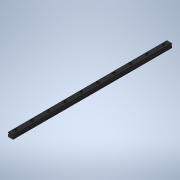
# Autodesk Inventor part: SSEB6-145-B3_r
Saved by Autodesk Inventor 2021 (Build 250183000, 183)
## iProperties
Created: 2025-06-10
Part Number: SSEB6-145-B3_r
Material: Generic
Catalog Web Link: www.cadenas.de
Description: SSEB, SSEB-MX, SSEBV, SSEBV-MX, SSE2B, SSE2B-MX, SSE2BV, SSE2BV-MX, SSEBL, SSEBL-MX, SSEBLV, SSEBLV-MX, SSE2BL, SSE2BL-MX, SSE2BLV, SSE2BLV-MX, SEB, SEBV, SE2B, SE2BV, SEBL, SEBLV, SE2BL, SE2BLV_rail-Miniature Linear Guides - Short Block, Standard Preload - High/Precision Grade
Vendor: MISUMI
Document SubType Name: Modeling
Designer: psAdmin
Manufacturer: MISUMI
Mass: 2.44458 g
Surface Area: 32.5102 cm^2
Volume: 2.44458 cm^3
Density: 1 g/cm^3
Appearance: PSOLRGB-175-175-175
Category: PARTsolutions
Company: MISUMI
Title: SSEB6-145-B3
Author: Cadenas PARTsolutions
Comments: Miniature Linear Guides - Short Block, Standard Preload - High/Precision Grade
PSOL_IDENT_0: {$CADENAS_DATA/23d-libs/misumi/metric/06_linear_guides/seb_series/seb_rail.prj},398 {VTYP=3D},{NB=SS
PSOL_IDENT_1: EB6-145-B3_r},{LINA=SSEB6-145-B3},{NN=SSEB, SSEB-MX, SSEBV, SSEBV-MX, SSE2B, SSE2B-MX, SSE2BV, SSE2B
PSOL_IDENT_2: V-MX, SSEBL, SSEBL-MX, SSEBLV, SSEBLV-MX, SSE2BL, SSE2BL-MX, SSE2BLV, SSE2BLV-MX, SEB, SEBV, SE2B, S
PSOL_IDENT_3: E2BV, SEBL, SEBLV, SE2BL, SE2BLV_rail},{DATE=17.02.2022 00:32:34},{GEOMDATE=21.01.2022 00:02:30},{VE
PSOL_IDENT_4: RSION=},{LINEID=90},{WBVAR=TS,ST,MAT,MX,NOB,LT,LS,ALT1,ALT2,ALT4},{WBNUMERIC=LS}  {NB=SSEB6-145-B3_r
PSOL_IDENT_5: },{LINA=SSEB6-145-B3},{KT=DUMMY},{PN=SSEB6-145-B3},{RT=B},{TS=},{TS1=  '','Advanced'  },{TYPE=SSEB},
PSOL_IDENT_6: {ST=S},{MAT=S},{MX=},{MXALG= '','w/o MX(Lubrication unit)' },{NOB=},{H=6},{LT=Selectable},{LTALG='Se
PSOL_IDENT_7: lectable','Selectable','Configurable','Configurable'},{LS=145},{W=12},{L1=17.4},{B=8},{C=0},{S=M2X1.
PSOL_IDENT_8: 5},{L2=9.7},{K=4.5},{CBB=0.3},{W1=5},{W2=3.5},{H1=4.0},{CAA=0.3},{DD1DD2HH=2.4x3.5x1},{F=15},{G=5.0}
PSOL_IDENT_9: ,{DD1=2.400},{DD2=3.500},{HH=1.000},{ALT1=},{ALT1ALG='', 'w/o MC (Tapped Holes)', '-MC', 'with MC (T
PSOL_IDENT_10: apped Holes)'},{MC=M2.6},{MC1=2.6},{ALT2=},{ALT2L=0.0},{ALT2N=0},{M=10},{LL=},{L0=25,40,55,70,85,100
PSOL_IDENT_11: ,115,130,145},{REC1=   '','Not applicable'    },{ST1='S', 'w/o Surface Treatment'},{MAT2='S','Stainl
PSOL_IDENT_12: ess Steel'},{NL=32.867},{ALT4=-B3},{ALT4ALG= '','w/o (Additional Blocks)','-B3','with B3(3-Block Typ
PSOL_IDENT_13: e (Adds 2 blocks.))','-B4','with B4(4-Block Type (Adds 3 blocks.))' },{CA1=0.3},{CA2=0.3},{VA1=1.5},
PSOL_IDENT_14: {HA1=1.0},{HA2=5.1372},{WA1=1.2167},{WA2=0.5},{RA1=1.00},{POIA1=-0.1473},{NA1=9},{LSC=6.0},{MS=2.0}
NB: SSEB6-145-B3_r
NN: SSEB, SSEB-MX, SSEBV, SSEBV-MX, SSE2B, SSE2B-MX, SSE2BV, SSE2BV-MX, SSEBL, SSEBL-MX, SSEBLV, SSEBLV-MX, SSE2BL, SSE2BL-MX, SSE2BLV, SSE2BLV-MX, SEB, SEBV, SE2B, SE2BV, SEBL, SEBLV, SE2BL, SE2BLV_rail
NT: Miniature Linear Guides - Short Block, Standard Preload - High/Precision Grade
NBSYN: $PN._r
LINA: SSEB6-145-B3
CATALOG: Misumi
PN: SSEB6-145-B3
TS: Advanced
ST: w/o Surface Treatment
MAT: Stainless Steel
MX: w/o MX(Lubrication unit)
NOB: 1
H: 6
LT: Selectable
LS: 145
W: 12
L1: 17.4
B: 8
C: 0
S: M2X1.5
L2: 9.7
K: 4.5
CBB: 0.3
W1: 5
W2: 3.5
H1: 4
CAA: 0.3
DD1DD2HH: 2.4x3.5x1
F: 15
G: 5
ALT1: w/o MC (Tapped Holes)
ALT2: Not applicable
ALT4: with B3(3-Block Type (Adds 2 blocks.))
NA1: 9
SUPPLIER: MISUMI
ARTICLENO: SSEB6-145-B3_r
BOMINFO: SSEB6-145-B3
CREATOR: CADENAS GmbH
Autodesk Inventor part; units mm, degrees
sketch "Sketch_12" plane through (0, 0, 0) normal (0, 0, 1) x (1, 0, 0)
  line L0 (-2.5, 3.7) -> (-2.5, 3.1084)
  line L1 (-2.5, 3.1084) -> (-2.3242, 3.0098)
  arc A0 (-2.1007, 2.75) -> (-2.3242, 3.0098) centre (-2.5686, 2.5736) ccw
  line L2 (-2.1007, 2.75) -> (-1.5, 2.75)
  line L3 (-1.5, 2.75) -> (-1.5, 2.25)
  line L4 (-1.5, 2.25) -> (-2.1007, 2.25)
  arc A1 (-2.3242, 1.9902) -> (-2.1007, 2.25) centre (-2.5686, 2.4264) ccw
  line L5 (-2.3242, 1.9902) -> (-2.5, 1.8917)
  line L6 (-2.5, 1.8917) -> (-2.5, 0.3)
  line L7 (-2.5, 0.3) -> (-2.2, 0)
  line L8 (-2.2, 0) -> (2.2, 0)
  line L9 (2.2, 0) -> (2.5, 0.3)
  line L10 (2.5, 0.3) -> (2.5, 1.8917)
  line L11 (2.5, 1.8917) -> (2.3242, 1.9902)
  arc A2 (2.1007, 2.25) -> (2.3242, 1.9902) centre (2.5686, 2.4263) ccw
  line L12 (2.1007, 2.25) -> (1.5, 2.25)
  line L13 (1.5, 2.25) -> (1.5, 2.75)
  line L14 (1.5, 2.75) -> (2.1007, 2.75)
  arc A3 (2.3242, 3.0098) -> (2.1007, 2.75) centre (2.5686, 2.5737) ccw
  line L15 (2.3242, 3.0098) -> (2.5, 3.1084)
  line L16 (2.5, 3.1084) -> (2.5, 3.7)
  line L17 (2.5, 3.7) -> (2.2, 4)
  line L18 (2.2, 4) -> (-2.2, 4)
  line L19 (-2.2, 4) -> (-2.5, 3.7)
  constraints: 40 end point, 8 point on circle, 4 centre point
extrude "Extrusion1" add sketch "Sketch_12" along normal mid plane 145
sketch "Sketch2" plane through (-2.2, 4, 72.5) normal (0, 1, 0) x (1, 0, 0)
  point P0 (2.2, 140)
hole "Hole1" at (0, 4, -67.5) direction (0, -1, 0) diameter 2.4 depth 4 counterbore diameter 3.5 counterbore depth 1
pattern_linear "Rectangular Pattern1" count 10 spacing 15 along (0, 0, 1) of "Hole1"
ref_plane "rail_to_adjusting_block_XY" through (0, 0, -67.5) normal (0, 1, 0) x (1, 0, 0)
ref_plane "rail_to_adjusting_block_YZ" through (0, 0, -67.5) normal (1, 0, 0) x (0, 0, -1)
ref_plane "rail_to_adjusting_block_ZX" through (0, 0, -67.5) normal (0, 0, -1) x (0, 1, 0)
ref_plane "screw_1_XY" through (0, 3, 67.5) normal (0, -1, 0) x (1, 0, 0)
ref_plane "screw_1_YZ" through (0, 3, 67.5) normal (1, 0, 0) x (0, 0, 1)
ref_plane "screw_1_ZX" through (0, 3, 67.5) normal (0, 0, 1) x (0, -1, 0)
ref_plane "screw_10_XY" through (0, 3, -67.5) normal (0, -1, 0) x (1, 0, 0)
ref_plane "screw_10_YZ" through (0, 3, -67.5) normal (1, 0, 0) x (0, 0, 1)
ref_plane "screw_10_ZX" through (0, 3, -67.5) normal (0, 0, 1) x (0, -1, 0)
ref_plane "screw_2_XY" through (0, 3, 52.5) normal (0, -1, 0) x (1, 0, 0)
ref_plane "screw_2_YZ" through (0, 3, 52.5) normal (1, 0, 0) x (0, 0, 1)
ref_plane "screw_2_ZX" through (0, 3, 52.5) normal (0, 0, 1) x (0, -1, 0)
ref_plane "screw_3_XY" through (0, 3, 37.5) normal (0, -1, 0) x (1, 0, 0)
ref_plane "screw_3_YZ" through (0, 3, 37.5) normal (1, 0, 0) x (0, 0, 1)
ref_plane "screw_3_ZX" through (0, 3, 37.5) normal (0, 0, 1) x (0, -1, 0)
ref_plane "screw_4_XY" through (0, 3, 22.5) normal (0, -1, 0) x (1, 0, 0)
ref_plane "screw_4_YZ" through (0, 3, 22.5) normal (1, 0, 0) x (0, 0, 1)
ref_plane "screw_4_ZX" through (0, 3, 22.5) normal (0, 0, 1) x (0, -1, 0)
ref_plane "screw_5_XY" through (0, 3, 7.5) normal (0, -1, 0) x (1, 0, 0)
ref_plane "screw_5_YZ" through (0, 3, 7.5) normal (1, 0, 0) x (0, 0, 1)
ref_plane "screw_5_ZX" through (0, 3, 7.5) normal (0, 0, 1) x (0, -1, 0)
ref_plane "screw_6_XY" through (0, 3, -7.5) normal (0, -1, 0) x (1, 0, 0)
ref_plane "screw_6_YZ" through (0, 3, -7.5) normal (1, 0, 0) x (0, 0, 1)
ref_plane "screw_6_ZX" through (0, 3, -7.5) normal (0, 0, 1) x (0, -1, 0)
ref_plane "screw_7_XY" through (0, 3, -22.5) normal (0, -1, 0) x (1, 0, 0)
ref_plane "screw_7_YZ" through (0, 3, -22.5) normal (1, 0, 0) x (0, 0, 1)
ref_plane "screw_7_ZX" through (0, 3, -22.5) normal (0, 0, 1) x (0, -1, 0)
ref_plane "screw_8_XY" through (0, 3, -37.5) normal (0, -1, 0) x (1, 0, 0)
ref_plane "screw_8_YZ" through (0, 3, -37.5) normal (1, 0, 0) x (0, 0, 1)
ref_plane "screw_8_ZX" through (0, 3, -37.5) normal (0, 0, 1) x (0, -1, 0)
ref_plane "screw_9_XY" through (0, 3, -52.5) normal (0, -1, 0) x (1, 0, 0)
ref_plane "screw_9_YZ" through (0, 3, -52.5) normal (1, 0, 0) x (0, 0, 1)
ref_plane "screw_9_ZX" through (0, 3, -52.5) normal (0, 0, 1) x (0, -1, 0)
ref_plane "to_block_XY" through (0, 4, 32.867) normal (0, 0, 1) x (1, 0, 0)
ref_plane "to_block_YZ" through (0, 4, 32.867) normal (1, 0, 0) x (0, 1, 0)
ref_plane "to_block_ZX" through (0, 4, 32.867) normal (0, 1, 0) x (0, 0, 1)
ref_plane "to_block_2_XY" through (0, 4, -32.867) normal (0, 0, 1) x (1, 0, 0)
ref_plane "to_block_2_YZ" through (0, 4, -32.867) normal (1, 0, 0) x (0, 1, 0)
ref_plane "to_block_2_ZX" through (0, 4, -32.867) normal (0, 1, 0) x (0, 0, 1)
ref_plane "to_block_3_XY" through (0, 4, 0) normal (0, 0, 1) x (1, 0, 0)
ref_plane "to_block_3_YZ" through (0, 4, 0) normal (1, 0, 0) x (0, 1, 0)
ref_plane "to_block_3_ZX" through (0, 4, 0) normal (0, 1, 0) x (0, 0, 1)
ref_plane "to_kue_XY" through (0, 0, 0) normal (0, 1, 0) x (1, 0, 0)
ref_plane "to_kue_YZ" through (0, 0, 0) normal (1, 0, 0) x (0, 0, -1)
ref_plane "to_kue_ZX" through (0, 0, 0) normal (0, 0, -1) x (0, 1, 0)
body "Solid1"
